pin_servo_gate (Autodesk Fusion 360 design; units mm, degrees)
Autodesk Fusion 360 part; units mm, degrees
sketch "Sketch1" plane through (0, 0, 0) normal (0, 0, 1) x (1, 0, 0)
  line L0 (0, -1.5) -> (3.8, -1.5)
  arc A0 (3.8, -1.5) -> (3.8, 1.5) centre (3.8, 0) ccw
  line L1 (3.8, 1.5) -> (0, 1.5)
  arc A1 (0, 1.5) -> (0, -1.5) centre (0, 0) ccw
  line L2 (0, 0) -> (3.8, 0) construction
  circle A2 centre (0, 0) radius 0.45
  circle A3 centre (3.8, 0) radius 0.45
  line L3 (0, -7) -> (3.8, -7)
  arc A4 (3.8, -7) -> (3.8, -4) centre (3.8, -5.5) ccw
  line L4 (3.8, -4) -> (0, -4)
  arc A5 (0, -4) -> (0, -7) centre (0, -5.5) ccw
  line L5 (0, -5.5) -> (3.8, -5.5) construction
  circle A6 centre (0, -5.5) radius 0.5
  circle A7 centre (3.8, -5.5) radius 0.5
  dimension "d1" = 3
  dimension "d2" = 0.9
  dimension "d3" = 0.9
  dimension "d8" = 3
  dimension "d9" = 1
  dimension "d10" = 1
  constraint tangent L0 A0
  constraint tangent A0 L1
  constraint parallel L0 L1
  constraint tangent L1 A1
  constraint tangent L0 A1
  constraint horizontal L2
  constraint coincident A1.centre L2.start
  constraint concentric A0 A3
  constraint tangent L3 A4
  constraint tangent A4 L4
  constraint parallel L3 L4
  constraint tangent L4 A5
  constraint tangent L3 A5
  constraint parallel L0 L5
  constraint concentric A5 A6
  constraint concentric A4 A7
  measures "d1" diameter of A0
  measures "d2" diameter of A2
  measures "d3" diameter of A3
  measures "d8" diameter of A4
  measures "d9" diameter of A6
  measures "d10" diameter of A7
extrude "Extrude1" add sketch "Sketch1" along normal blind 4 contours A2 | A3 makes body 1 at (0.4494, -0.0224, 2.6667) makes body 2 at (4.2494, -0.0224, 2.6667)
extrude "Extrude2" add sketch "Sketch1" against normal blind 1 separate body contours L0 A0 L1 A1 | A2 | A3 makes body 3
extrude "Extrude3" add sketch "Sketch1" against normal blind 1 separate body contours L3 A4 L4 A5 makes body 4
